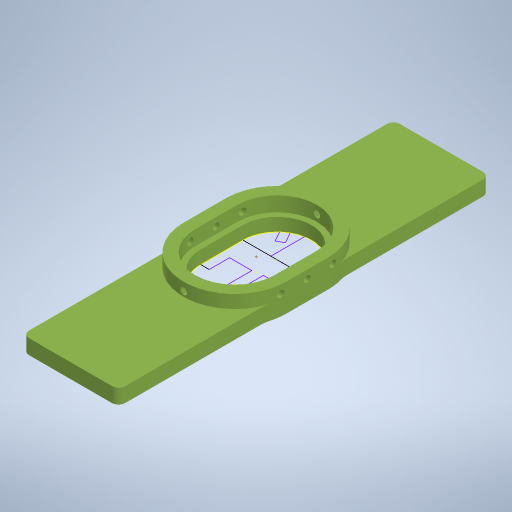
# Autodesk Inventor part: holder_base
Saved by Autodesk Inventor 2024 (Build 280153000, 153)
## iProperties
Created: 2023-06-16
Part Number: holder_base
Material: Generic
Document SubType Name: Modeling
Designer: Rober
Density: 1 g/cm^3
Appearance: Olive Green
Mass: 11.7985 g
Surface Area: 67.7673 cm^2
Volume: 11.7985 cm^3
Author: Rober
Autodesk Inventor part; units mm, degrees
ref_plane "YZ Plane" through (0, 0, 0) normal (1, 0, 0) x (0, 1, 0)
ref_plane "XZ Plane" through (0, 0, 0) normal (0, 1, 0) x (-1, 0, 0)
ref_plane "XY Plane" through (0, 0, 0) normal (0, 0, 1) x (1, 0, 0)
sketch "Chamber_outline" plane through (0, 0, 0) normal (0, 1, 0) x (-1, 0, 0)
  line L0 (0, -6.495) -> (0, 6.495) construction
  line L1 (12.185, -6.495) -> (12.185, 6.495)
  line L2 (-12.185, 6.495) -> (-12.185, -6.495)
  arc A0 (-12.185, -6.495) -> (12.185, -6.495) centre (0, -6.495) ccw
  arc A1 (12.185, 6.495) -> (-12.185, 6.495) centre (0, 6.495) ccw
  line L3 (15.7049, -6.495) -> (15.7049, 6.495)
  arc A2 (15.7049, 6.495) -> (-15.7049, 6.495) centre (0, 6.495) ccw
  line L4 (-15.7049, 6.495) -> (-15.7049, -6.495)
  arc A3 (-15.7049, -6.495) -> (15.7049, -6.495) centre (0, -6.495) ccw
  line L5 (12.185, 0) -> (-12.185, 0)
  line L6 (14.7497, -11.8886) -> (14.7497, -56.8886)
  line L7 (14.7497, -56.8886) -> (-14.7497, -56.8886)
  line L8 (-14.7497, -56.8886) -> (-14.7497, -11.8886)
  line L9 (14.7497, 11.8886) -> (14.7497, 56.8886)
  line L10 (14.7497, 56.8886) -> (-14.7497, 56.8886)
  line L11 (-14.7497, 56.8886) -> (-14.7497, 11.8886)
  line L12 (10.485, -6.495) -> (10.485, 6.495)
  arc A4 (10.485, 6.495) -> (-10.485, 6.495) centre (0, 6.495) ccw
  line L13 (-10.485, 6.495) -> (-10.485, -6.495)
  arc A5 (-10.485, -6.495) -> (10.485, -6.495) centre (0, -6.495) ccw
  point P0 (0, 0)
  point P1 (0, 0)
  point P2 (0, 0)
  point P3 (0, -56.8886)
  point P4 (0, 56.8886)
  point P5 (-14.7497, 11.8886)
  point P6 (14.7497, 11.8886)
  point P7 (0, -18.68)
  point P8 (0, 18.68)
  dimension "d18" = 24.37
  dimension "d26" = 1.7
  dimension "d58" = 45
  dimension "d82" = 37.36
  constraints: 30 end point, 16 point on circle, 6 centre point, 5 midpoint, 5 symmetric about line, 4 parallel, 4 tangent, 3 perpendicular, 1 coincident, 1 vertical, 6 other
  measures "d18" distance between parallel lines of L2 L1
  measures "d26" radial gap between concentric circles of A0 A5
  measures "d58" distance of L10.end L11.end
  measures "d82" distance of point (0, -18.68) point (0, 18.68)
extrude "Extrusion3" add sketch "Chamber_outline" along normal blind 4.5 contours A3 L4 A2 L3
extrude "Extrusion4" add sketch "Chamber_outline" along normal blind 0.5 contours L6 L7 L8 A3 | A2 L11 L10 L9
extrude "Extrusion5" add sketch "Chamber_outline" against normal blind 4 contours A0 L2 L5 L13 A5 L12 L1 | L5 L12 A4 L13 L2 A1 L1 | A3 L4 A2 L3 | L6 L7 L8 A3 | A2 L11 L10 L9
fillet "Fillet1" radius 10 2 edges at (-14.7497, -2, 11.8886) (-14.7497, 0.25, 11.8886)
fillet "Fillet2" radius 10 6 edges at (-14.7497, -2, -11.8886) (-14.7497, 0.25, -11.8886) (14.7497, 0.25, -11.8886) (14.7497, -2, -11.8886) (14.7497, 0.25, 11.8886) (14.7497, -2, 11.8886)
fillet "Fillet3" radius 2 8 edges at (-14.7497, -2, -56.8886) (-14.7497, 0.25, -56.8886) (-14.7497, -2, 56.8886) (-14.7497, 0.25, 56.8886) (14.7497, -2, 56.8886) (14.7497, 0.25, 56.8886) (14.7497, -2, -56.8886) (14.7497, 0.25, -56.8886)
sketch "Sketch9" plane through (0, -4, 0) normal (0, -1, 0) x (1, 0, 0)
  line L0 (0.801, 42.3276) -> (0.801, 45.3727) construction
  line L1 (0.801, 45.3727) -> (3.851, 45.3727) construction
  line L2 (3.851, 45.3727) -> (3.851, 42.3276) construction
  line L3 (3.851, 42.3276) -> (0.801, 42.3276) construction
  line L4 (10.801, 43.349) -> (0.801, 43.349)
  line L5 (0.801, 43.349) -> (0.801, 47.602)
  spline S0 degree 2 poles (0.801, 47.602) (0.801, 49.2102) (1.3422, 50.6584) (2.7141, 51.5349) (3.6059, 51.5349) knots 0 0 0 1 2 3 3 3
  spline S1 degree 2 poles (3.6059, 51.5349) (4.7263, 51.5349) (6.1973, 50.2163) (6.3879, 48.8977) knots 0 0 0 1 2 2 2
  spline S2 degree 2 poles (6.3879, 48.8977) (6.769, 49.5532) (7.6836, 50.4069) (8.8498, 51.131) knots 0 0 0 1 2 2 2
  line L6 (8.8498, 51.131) -> (10.801, 52.3505)
  line L7 (10.801, 52.3505) -> (10.801, 49.9343)
  line L8 (10.801, 49.9343) -> (8.6211, 48.4785)
  spline S3 degree 2 poles (8.6211, 48.4785) (7.455, 47.6935) (6.8452, 47.1218) (6.6242, 46.4816) (6.6242, 45.7804) knots 0 0 0 1 2 3 3 3
  line L9 (6.6242, 45.7804) -> (6.6242, 45.3688)
  line L10 (6.6242, 45.3688) -> (10.801, 45.3688)
  line L11 (10.801, 45.3688) -> (10.801, 43.349)
  line L12 (5.0312, 45.3688) -> (5.0312, 46.8627)
  spline S4 degree 2 poles (5.0312, 46.8627) (5.0312, 48.3185) (4.7873, 49.0426) (4.1851, 49.4541) (3.7355, 49.4541) knots 0 0 0 1 2 3 3 3
  spline S5 degree 2 poles (3.7355, 49.4541) (3.2324, 49.4541) (2.6074, 48.913) (2.5236, 48.4252) knots 0 0 0 1 2 2 2
  spline S6 degree 2 poles (2.5236, 48.4252) (2.4931, 48.1737) (2.4931, 46.9465) knots 0 0 0 1 1 1
  line L13 (2.4931, 46.9465) -> (2.4931, 45.3688)
  line L14 (2.4931, 45.3688) -> (5.0312, 45.3688)
  point P0 (0, 0)
  constraints: 2 other
extrude "Extrusion14" cut sketch "Sketch9" against normal blind 2
sketch "Sketch3" plane through (15.7049, 4.5, 6.495) normal (1, 0, 0) x (0, 0, -1)
  circle A0 centre (6.5, -2.5) radius 1
  line L0 (0, 0) -> (12.99, 0) projected
  circle A1 centre (14.5, -2.5) radius 1
  circle A2 centre (-1.5, -2.5) radius 1
  point P0 (6.495, -4.5)
  dimension "d41" = 2
  dimension "d43" = 2.5
  dimension "d85" = 2
  dimension "d86" = 2
  dimension "d87" = 8
  dimension "d88" = 8
  constraints: 3 centre point
  measures "d41" diameter of A0
  measures "d43" distance from line of L0 A0.centre
  measures "d85" diameter of A1
  measures "d86" diameter of A2
  measures "d87" distance of A0.centre A2.centre
  measures "d88" distance of A1.centre A0.centre
extrude "Extrusion6" cut sketch "Sketch3" against normal through all
sketch "Sketch4" plane through (-12.7497, 0.5, 56.8886) normal (0, 0, 1) x (1, 0, 0)
  circle A0 centre (12.7497, 1.5) radius 1
  line L0 (28.4546, 4) -> (-2.9552, 4) projected
  point P0 (12.7497, -0.5)
  point P1 (12.7497, 4)
  dimension "d36" = 2
  dimension "d42" = 2.5
  constraints: 1 centre point, 1 midpoint
  measures "d36" diameter of A0
  measures "d42" distance of point (12.75, 4) A0.centre
extrude "Extrusion7" cut sketch "Sketch4" against normal through all
sketch "Sketch5" plane through (0, -4, 0) normal (0, -1, 0) x (1, 0, 0)
  line L0 (-10.485, -6.495) -> (-10.485, 6.495) projected
  line L1 (-10.485, -6.495) -> (-8.4271, -6.495)
  line L2 (-7.9121, 0.245) -> (-7.9121, 6.495)
  line L3 (-7.9121, 6.495) -> (-10.485, 6.495)
  line L4 (10.485, -6.495) -> (10.485, 6.495) projected
  line L5 (10.485, -6.495) -> (8.4271, -6.495)
  line L6 (8.3305, -0.2609) -> (8.3305, 6.495)
  line L7 (8.3305, 6.495) -> (10.485, 6.495)
  arc A0 (10.485, 6.495) -> (-10.485, 6.495) centre (0, 6.495) ccw projected
  arc A1 (-10.485, -6.495) -> (10.485, -6.495) centre (0, -6.495) ccw projected
  arc A2 (-10.485, -6.495) -> (10.485, -6.495) centre (0, -6.495) ccw projected
  line L8 (-7.079, -14.2295) -> (-5.3711, -11.1831)
  line L9 (-5.3711, -11.1831) -> (-3.3516, -12.3154)
  line L10 (-3.3516, -12.3154) -> (-5.1945, -15.6028)
  line L11 (-7.4267, 14.3644) -> (-5.7188, 11.3181)
  line L12 (-5.7188, 11.3181) -> (-3.6001, 12.5059)
  line L13 (-3.6001, 12.5059) -> (-5.4497, 15.8051)
  line L14 (3.586, 12.9764) -> (5.1976, 15.6011)
  line L15 (5.8011, 11.7346) -> (3.586, 12.9764)
  line L16 (7.1611, 14.1536) -> (5.8011, 11.7346)
  line L17 (-10.485, -6.495) -> (10.8395, -6.495)
  line L18 (1.9666, 16.7939) -> (1.9666, -0.2609)
  line L19 (-2.0003, -16.7874) -> (-2.0003, -6.495)
  line L20 (-1.0812, 0.245) -> (-1.0812, 16.9241)
  line L21 (4.8643, -15.7834) -> (4.8643, -6.495)
  line L22 (-7.9121, 0.245) -> (-1.0812, 0.245)
  line L23 (1.9666, -0.2609) -> (8.3305, -0.2609)
  point P0 (0, 0)
  point P1 (1.5355, -6.495)
  point P2 (-7.079, -14.2295)
  point P3 (-5.1945, -15.6028)
  point P4 (-5.3016, 15.5409)
  point P5 (-7.2574, 14.0624)
  point P6 (7.5128, 14.2848)
  point P7 (5.4529, 15.8033)
  point P8 (8.4271, -6.495)
  point P9 (4.8643, -15.7834)
  constraints: 44 end point, 8 point on circle, 7 perpendicular, 4 point on line, 3 horizontal, 3 vertical, 1 collinear, 1 parallel
sketch "Sketch6" plane through (0, -4, 0) normal (0, -1, 0) x (1, 0, 0)
  ellipse E0 centre (0, -5) end of major axis (0.355, -4.9802) minor radius 0.3556 projected
  circle A0 centre (1, -5.9999) radius 0.3556 projected
  circle A1 centre (0, -5.9999) radius 0.3556 projected
  circle A2 centre (-1, -6) radius 0.3556 projected
  circle A3 centre (-1, -4.9999) radius 0.3556 projected
  circle A4 centre (1, -5) radius 0.3556 projected
  circle A5 centre (1, -6.9999) radius 0.3556 projected
  ellipse E1 centre (0, -7) end of major axis (0.3551, -6.9801) minor radius 0.3556 projected
  ellipse E2 centre (-1, -7) end of major axis (-0.645, -6.9801) minor radius 0.3556 projected
  ellipse E3 centre (6, -3) end of major axis (6.355, -2.9802) minor radius 0.3556 projected
  circle A6 centre (5, -3) radius 0.3556 projected
  ellipse E4 centre (4, -2.9999) end of major axis (4.3551, -2.9801) minor radius 0.3556 projected
  circle A7 centre (4, -4) radius 0.3556 projected
  ellipse E5 centre (5, -4) end of major axis (5.355, -3.9802) minor radius 0.3556 projected
  ellipse E6 centre (6, -3.9999) end of major axis (6.3551, -3.9801) minor radius 0.3556 projected
  circle A8 centre (6, -2) radius 0.3556 projected
  circle A9 centre (5, -2) radius 0.3556 projected
  circle A10 centre (4, -1.9999) radius 0.3556 projected
  circle A11 centre (3, -12) radius 0.3556 projected
  circle A12 centre (4, -11.9999) radius 0.3556 projected
  circle A13 centre (3, -10.9999) radius 0.3556 projected
  circle A14 centre (4, -11) radius 0.3556 projected
  circle A15 centre (2, -10.9999) radius 0.3556 projected
  circle A16 centre (2, -12) radius 0.3556 projected
  circle A17 centre (2, -13) radius 0.3555 projected
  ellipse E7 centre (3, -13) end of major axis (3.0198, -13.355) minor radius 0.3556 projected
  ellipse E8 centre (4, -13) end of major axis (4.0198, -13.355) minor radius 0.3556 projected
  circle A18 centre (1.5, 9) radius 0.3556 projected
  circle A19 centre (1.5, 8) radius 0.3556 projected
  circle A20 centre (0.5, 8) radius 0.3556 projected
  ellipse E9 centre (-0.5, 8.0001) end of major axis (-0.1449, 8.0199) minor radius 0.3556 projected
  circle A21 centre (-0.5, 9) radius 0.3556 projected
  circle A22 centre (-0.5, 10) radius 0.3556 projected
  circle A23 centre (1.5, 10.0001) radius 0.3556 projected
  ellipse E10 centre (0.5, 10) end of major axis (0.5198, 9.645) minor radius 0.3556 projected
  circle A24 centre (0.5, 9) radius 0.3556 projected
  circle A25 centre (3, -12) radius 0.4056
  circle A26 centre (0, -5.9999) radius 0.4056
  circle A27 centre (5, -3) radius 0.4056
  circle A28 centre (0.5, 9) radius 0.4056
  circle A29 centre (-1, -6) radius 0.4056
  point P0 (0, 0)
  dimension "d63" = 0.05
  dimension "d64" = 0.05
  dimension "d65" = 0.05
  dimension "d66" = 0.05
  dimension "d77" = 0.05
  constraints: 5 centre point
  measures "d63" radial gap between concentric circles of A11 A25
  measures "d64" radial gap between concentric circles of A1 A26
  measures "d65" radial gap between concentric circles of A6 A27
  measures "d66" radial gap between concentric circles of A24 A28
  measures "d77" radial gap between concentric circles of A2 A29
sketch "Sketch7" plane through (0, -0.5, 0) normal (0, 1, 0) x (1, 0, 0)
  arc A0 (12.185, 6.495) -> (-12.185, 6.495) centre (0, 6.495) ccw projected
  arc A1 (10.285, 6.495) -> (-10.285, 6.495) centre (0, 6.495) ccw
  line L0 (-10.485, -6.495) -> (-10.485, 6.495) projected
  arc A2 (10.485, 6.495) -> (-10.485, 6.495) centre (0, 6.495) ccw projected
  line L1 (10.485, 6.495) -> (10.485, -6.495) projected
  arc A3 (-10.485, -6.495) -> (10.485, -6.495) centre (0, -6.495) ccw projected
  line L2 (-12.185, -6.495) -> (-12.185, 6.495) projected
  arc A4 (-12.185, -6.495) -> (12.185, -6.495) centre (0, -6.495) ccw projected
  line L3 (12.185, 6.495) -> (12.185, -6.495) projected
  arc A5 (12.185, 6.495) -> (-12.185, 6.495) centre (0, 6.495) ccw projected
  arc A6 (-12.185, -6.495) -> (12.185, -6.495) centre (0, -6.495) ccw projected
  line L4 (12.185, 6.495) -> (12.185, -6.495) projected
  line L5 (-12.185, -6.495) -> (-12.185, 6.495) projected
  line L6 (-10.285, -6.495) -> (-10.285, 6.495)
  arc A7 (10.285, 6.495) -> (-10.285, 6.495) centre (0, 6.495) ccw
  line L7 (10.285, 6.495) -> (10.285, -6.495)
  arc A8 (-10.285, -6.495) -> (10.285, -6.495) centre (0, -6.495) ccw
  circle A9 centre (5, 3) radius 0.4056 projected
  circle A10 centre (0, 5.9999) radius 0.4056 projected
  circle A11 centre (0.5, -9) radius 0.4056 projected
  circle A12 centre (3, 12) radius 0.4056 projected
  line L8 (10.485, 6.495) -> (4.8643, 6.495) projected
  line L9 (4.8643, 6.495) -> (4.8643, 15.7834) projected
  arc A13 (4.8643, 15.7834) -> (-2.0003, 16.7874) centre (0, 6.495) ccw projected
  line L10 (-2.0003, 16.7874) -> (-2.0003, 6.495) projected
  line L11 (-2.0003, 6.495) -> (-10.485, 6.495) projected
  line L12 (-10.485, -6.495) -> (-10.485, 6.495) projected
  line L13 (-10.485, -6.495) -> (-7.9121, -6.495) projected
  line L14 (-7.9121, -6.495) -> (-7.9121, -0.245) projected
  line L15 (-7.9121, -0.245) -> (-1.0812, -0.245) projected
  line L16 (-1.0812, -0.245) -> (-1.0812, -16.9241) projected
  arc A14 (-1.0812, -16.9241) -> (1.9666, -16.7939) centre (0, -6.495) ccw projected
  line L17 (1.9666, -16.7939) -> (1.9666, 0.2609) projected
  line L18 (1.9666, 0.2609) -> (8.3305, 0.2609) projected
  line L19 (8.3305, 0.2609) -> (8.3305, -6.495) projected
  line L20 (8.3305, -6.495) -> (10.485, -6.495) projected
  line L21 (10.485, 6.495) -> (10.485, -6.495) projected
  line L22 (7.1611, -14.1536) -> (5.8011, -11.7346) projected
  line L23 (5.8011, -11.7346) -> (3.586, -12.9764) projected
  line L24 (3.586, -12.9764) -> (5.1976, -15.6011) projected
  arc A15 (5.1976, -15.6011) -> (7.1611, -14.1536) centre (0, -6.495) ccw projected
  line L25 (-7.079, 14.2295) -> (-5.3711, 11.1831) projected
  line L26 (-5.3711, 11.1831) -> (-3.3516, 12.3154) projected
  line L27 (-3.3516, 12.3154) -> (-5.1945, 15.6028) projected
  arc A16 (-5.1945, 15.6028) -> (-7.079, 14.2295) centre (0, 6.495) ccw projected
  line L28 (-5.3016, -15.5409) -> (-3.6001, -12.5059) projected
  line L29 (-3.6001, -12.5059) -> (-5.7188, -11.3181) projected
  line L30 (-5.7188, -11.3181) -> (-7.2574, -14.0624) projected
  arc A17 (-7.2574, -14.0624) -> (-5.3016, -15.5409) centre (0, -6.495) ccw projected
  circle A18 centre (-1, 6) radius 0.4056 projected
  line L31 (0, -16.78) -> (0, 0)
  line L32 (-10.285, 0) -> (0, 0)
  line L33 (0, 0) -> (10.285, 0)
  line L34 (0, 0) -> (0, 16.78)
  point P0 (-1.0812, -16.723)
  point P1 (1.9666, -16.5902)
  point P2 (10.285, -6.495)
  point P3 (10.285, 6.495)
  point P4 (4.8643, 15.557)
  point P5 (-2.0003, 16.5836)
  point P6 (-10.285, 6.495)
  point P7 (-10.285, -6.495)
  point P8 (5.0929, -15.4305)
  point P9 (7.0601, -13.974)
  point P10 (-7.1563, -13.8821)
  point P11 (-5.2037, -15.3664)
  point P12 (-5.0967, 15.4283)
  point P13 (-6.9785, 14.0503)
  dimension "d83" = 33.56
  constraints: 12 end point, 8 point on circle, 3 centre point, 2 midpoint, 2 perpendicular, 2 vertical, 1 collinear, 1 point on line, 2 other
  measures "d83" distance of L34.end L31.start
equation "\"metal_holder_thickness\" = 5"
equation "\"metal_holder_slot_length\" = 5"
body "Solid2"
